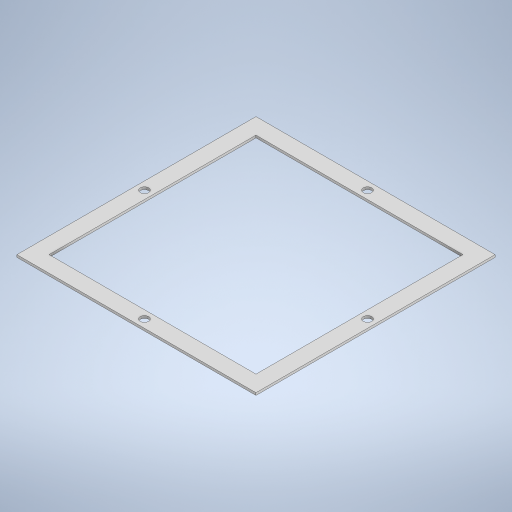
# Autodesk Inventor part: top plate
Saved by Autodesk Inventor 2024.2 (Build 282272000, 272)
## iProperties
Created: 2024-11-04
Part Number: top plate
Material: Generic
Document SubType Name: Modeling
Designer: Tom
Density: 1 g/cm^3
Appearance: Default
Author: Tom
Autodesk Inventor part; units mm, degrees
ref_plane "YZ Plane" through (0, 0, 0) normal (1, 0, 0) x (0, 1, 0)
ref_plane "XZ Plane" through (0, 0, 0) normal (0, 1, 0) x (-1, 0, 0)
ref_plane "XY Plane" through (0, 0, 0) normal (0, 0, 1) x (1, 0, 0)
sketch "Sketch1" plane through (0, 0, 0) normal (0, 1, 0) x (-1, 0, 0)
  line L0 (0, 0) -> (88.9, 0)
  line L1 (88.9, 0) -> (88.9, -88.9)
  line L2 (88.9, -88.9) -> (0, -88.9)
  line L3 (0, -88.9) -> (0, 0)
  line L4 (82.931, -5.969) -> (5.969, -5.969)
  line L5 (5.969, -5.969) -> (5.969, -82.931)
  line L6 (5.969, -82.931) -> (82.931, -82.931)
  line L7 (82.931, -82.931) -> (82.931, -5.969)
  point P0 (44.45, -5.969)
  dimension "d0" = 88.9
  dimension "d1" = 88.9
  dimension "d2" = 5.969
  dimension "d3" = 5.969
  dimension "d4" = 5.969
  dimension "d5" = 5.969
  constraints: 16 end point, 4 parallel, 2 horizontal, 2 perpendicular, 1 midpoint
  measures "d0" distance of L0.end L1.end
  measures "d1" distance of L0.start L0.end
  measures "d2" distance between parallel lines of L1 L7
  measures "d3" distance between parallel lines of L2 L6
  measures "d4" distance between parallel lines of L3 L5
  measures "d5" distance from line of L0 point (44.45, -5.969)
extrude "Extrusion1" add sketch "Sketch1" along normal blind 0.889
sketch "Sketch2" plane through (0, 0.889, 0) normal (0, 1, 0) x (1, 0, 0)
  circle A0 centre (-85.9155, 44.45) radius 1.5875
  line L0 (-88.9, 88.9) -> (-88.9, 0) projected
  line L1 (0, 88.9) -> (-88.9, 88.9) projected
  circle A1 centre (-2.9845, 44.45) radius 1.5875
  line L2 (-5.969, 82.931) -> (-5.969, 5.969) projected
  circle A2 centre (-44.45, 2.9845) radius 1.5875
  line L3 (-5.969, 5.969) -> (-82.931, 5.969) projected
  circle A3 centre (-44.45, 85.9155) radius 1.5875
  line L4 (-82.931, 82.931) -> (-5.969, 82.931) projected
  point P0 (0, 0)
  dimension "d8" = 3.175
  dimension "d9" = 2.9845
  dimension "d10" = 44.45
  dimension "d11" = 3.175
  dimension "d12" = 2.9845
  dimension "d13" = 3.175
  dimension "d14" = 2.9845
  dimension "d15" = 3.175
  dimension "d16" = 2.9845
  constraints: 4 centre point
  measures "d8" diameter of A0
  measures "d9" distance from line of L0 A0.centre
  measures "d10" distance from line of L1 A0.centre
  measures "d11" diameter of A1
  measures "d12" distance from line of L2 A1.centre
  measures "d13" diameter of A2
  measures "d14" distance from line of L3 A2.centre
  measures "d15" diameter of A3
  measures "d16" distance from line of L4 A3.centre
extrude "Extrusion2" cut sketch "Sketch2" against normal through all
body "Solid1"
